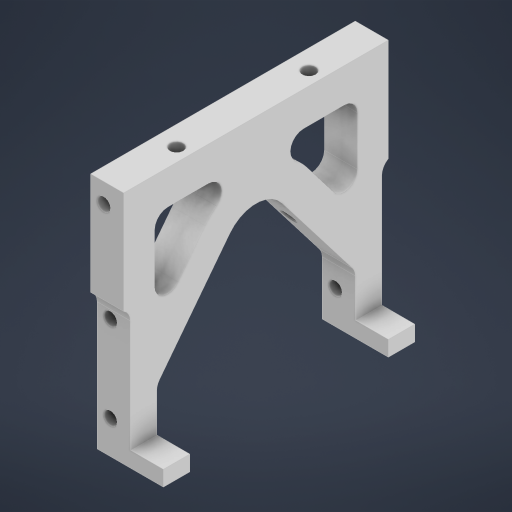
# Autodesk Inventor part: InsidePereborka
Saved by Autodesk Inventor 2024 (Build 280153000, 153)
## iProperties
Created: 2023-01-07
Part Number: InsidePereborka
Material: Типовые
Document SubType Name: Modeling
Designer: KirikDK
Density: 1 g/cm^3
Appearance: По умолчанию
Mass: 27.6494 g
Surface Area: 128.309 cm^2
Volume: 27.6494 cm^3
Author: KirikDK
Autodesk Inventor part; units mm, degrees
ref_plane "YZ Plane" through (0, 0, 0) normal (1, 0, 0) x (0, 1, 0)
ref_plane "XZ Plane" through (0, 0, 0) normal (0, 1, 0) x (-1, 0, 0)
ref_plane "XY Plane" through (0, 0, 0) normal (0, 0, 1) x (1, 0, 0)
sketch "Эскиз1" plane through (0, 0, 0) normal (1, 0, 0) x (0, 1, 0)
  line L0 (49.3333, 18.3333) -> (-26.6667, 18.3333)
  line L1 (-26.6667, 18.3333) -> (-26.6667, -61.6667)
  line L2 (-26.6667, -61.6667) -> (49.3333, -61.6667)
  line L3 (49.3333, -61.6667) -> (49.3333, 18.3333)
  line L4 (17.3333, 18.3333) -> (17.3333, 16.3333)
  line L5 (17.3333, 16.3333) -> (-24.6667, 16.3333)
  line L6 (-24.6667, 16.3333) -> (-24.6667, -21.6667)
  line L7 (-24.6667, -21.6667) -> (-26.6667, -21.6667)
  line L8 (17.3333, -61.6667) -> (17.3333, -59.6667)
  line L9 (17.3333, -59.6667) -> (-24.6667, -59.6667)
  line L10 (-24.6667, -59.6667) -> (-24.6667, -21.6667)
  line L11 (-24.6667, -21.6667) -> (-26.6667, -21.6667)
  line L12 (-24.6667, 8.3333) -> (-7, 8.3333)
  line L13 (-7, 8.3333) -> (-7, -51.6667)
  line L14 (-7, -51.6667) -> (-24.6667, -51.6667)
  line L15 (-24.6667, -51.6667) -> (-24.6667, 8.3333)
  line L16 (-7, 8.3333) -> (32, -21.6667)
  line L17 (32, -21.6667) -> (-7, -51.6667)
  point P0 (0, 0)
  point P1 (-24.6667, -51.6667)
  dimension "d0" = 80
  dimension "d1" = 2
  dimension "d2" = 2
  dimension "d3" = 2
  dimension "d4" = 2
  dimension "d5" = 44
  dimension "d6" = 44
  dimension "d7" = 40
  dimension "d8" = 40
  dimension "d9" = 76
  dimension "d10" = 10
  dimension "d11" = 10
  constraints: 36 end point, 8 perpendicular, 4 parallel, 3 point on line, 2 horizontal, 2 midpoint, 2 vertical
  measures "d0" distance of L2.end L0.start
  measures "d1" distance between parallel lines of L0 L5
  measures "d2" distance between parallel lines of L1 L6
  measures "d3" distance between parallel lines of L1 L10
  measures "d4" distance between parallel lines of L2 L9
  measures "d5" distance between parallel lines of L1 L8
  measures "d6" distance between parallel lines of L1 L4
  measures "d7" distance between parallel lines of L0 L7
  measures "d8" distance between parallel lines of L11 L2
  measures "d9" distance between parallel lines of L1 L3
  measures "d10" distance between parallel lines of L0 L12
  measures "d11" distance between parallel lines of L2 L14
extrude "Выдавливание1" add sketch "Эскиз1" along normal blind 10 contours L3 L2 L8 L9 L10 L14 L17 L16 L12 L6 L5 L4 L0
fillet "Сопряжение1" radius 10 1 edges at (5, 32, -21.6667)
fillet "Сопряжение3" radius 4 4 edges at (5, 17.3333, -59.6667) (5, 17.3333, 16.3333) (5, -7, -51.6667) (5, -7, 8.3333)
sketch "Эскиз2" plane through (10, 49.3333, -61.6667) normal (0, 0, -1) x (-1, 0, 0)
  circle A0 centre (6, -7) radius 2
  circle A1 centre (6, -38) radius 2
  circle A2 centre (6, -64) radius 2
  point P0 (10, -49.3333)
  constraints: 3 centre point
sketch "Эскиз3" plane through (0, 49.3333, 18.3333) normal (0, 1, 0) x (1, 0, 0)
  circle A0 centre (6, 60) radius 2
  circle A1 centre (6, 20) radius 2
  point P0 (0, 18.3333)
  constraints: 2 centre point
extrude "Выдавливание2" cut sketch "Эскиз2" against normal blind 100
extrude "Выдавливание3" cut sketch "Эскиз3" against normal blind 20
sketch "Эскиз4" plane through (10, 0, 0) normal (1, 0, 0) x (0, 0, -1)
  line L0 (59.6667, -24.6667) -> (59.6667, 13.8692) projected
  arc A0 (61.6667, 17.3333) -> (59.6667, 13.8692) centre (63.6667, 13.8692) ccw projected
  line L1 (61.6667, 17.3333) -> (61.6667, 49.3333) projected
  line L2 (61.6667, 49.3333) -> (-18.3333, 49.3333) projected
  line L3 (-18.3333, 49.3333) -> (-18.3333, 17.3333) projected
  arc A1 (-16.3333, 13.8692) -> (-18.3333, 17.3333) centre (-20.3333, 13.8692) ccw projected
  line L4 (-16.3333, 13.8692) -> (-16.3333, -24.6667) projected
  line L5 (-16.3333, -24.6667) -> (-8.3333, -24.6667) projected
  line L6 (-8.3333, -24.6667) -> (-8.3333, -8.3605) projected
  arc A2 (-7.5038, -5.9216) -> (-8.3333, -8.3605) centre (-4.3333, -8.3605) ccw projected
  line L7 (-7.5038, -5.9216) -> (13.7404, 21.6959) projected
  arc A3 (29.5929, 21.6959) -> (13.7404, 21.6959) centre (21.6667, 15.5988) ccw projected
  line L8 (29.5929, 21.6959) -> (50.8372, -5.9216) projected
  arc A4 (51.6667, -8.3605) -> (50.8372, -5.9216) centre (47.6667, -8.3605) ccw projected
  line L9 (51.6667, -8.3605) -> (51.6667, -24.6667) projected
  line L10 (51.6667, -24.6667) -> (59.6667, -24.6667) projected
  line L11 (-9, 7.4411) -> (-9, 40)
  line L12 (-9, 40) -> (52.3333, 40)
  line L13 (52.3333, 40) -> (52.3333, 7.4411)
  line L14 (52.3333, 7.4411) -> (36.9907, 27.3865)
  arc A5 (36.9907, 27.3865) -> (6.3426, 27.3865) centre (21.6667, 15.5988) ccw
  line L15 (6.3426, 27.3865) -> (-9, 7.4411)
  point P0 (0, 0)
  constraints: 10 end point, 2 point on circle, 1 centre point, 5 other
extrude "Выдавливание4" cut sketch "Эскиз4" against normal blind 22 contours L11 L12 L13 L14 A5 L15
sketch "Эскиз5" plane through (10, 0, 0) normal (1, 0, 0) x (0, 0, -1)
  line L0 (11.6667, 43) -> (31.6667, 43)
  line L1 (31.6667, 43) -> (31.6667, 31)
  line L2 (31.6667, 31) -> (11.6667, 31)
  line L3 (11.6667, 31) -> (11.6667, 43)
  line L4 (61.6667, 17.3333) -> (61.6667, 49.3333) projected
  line L5 (-18.3333, 49.3333) -> (-18.3333, 17.3333) projected
  line L6 (-11, 40) -> (55, 40)
  line L7 (55, 40) -> (55, 38)
  line L8 (55, 38) -> (-11, 38)
  line L9 (-11, 38) -> (-11, 40)
  line L10 (52.3333, 7.4411) -> (44.4016, 17.7523)
  line L11 (52.3333, 7.4411) -> (36.9907, 27.3865) projected
  line L12 (44.4016, 17.7523) -> (41, 14)
  line L13 (41, 14) -> (54.2371, 2)
  line L14 (54.2371, 2) -> (54.6936, 25.6036)
  line L15 (54.6936, 25.6036) -> (52.3333, 23)
  line L16 (52.3333, 13.3333) -> (52.3333, 9.3333) projected
  line L17 (52.3333, 40) -> (52.3333, 7.4411) projected
  line L18 (52.3333, 23) -> (52.3333, 7.4411)
  line L19 (-9, 7.4411) -> (6.3426, 27.3865) projected
  line L20 (1.5689, 21.1808) -> (4, 19)
  line L21 (4, 19) -> (-11, 1.3744)
  line L22 (-11, 1.3744) -> (-11, 26)
  line L23 (-11, 26) -> (-9, 26)
  line L24 (-9, 7.4411) -> (-9, 40) projected
  line L25 (1.5689, 21.1808) -> (-9, 7.4411)
  line L26 (-9, 7.4411) -> (-9, 26)
  point P0 (0, 0)
  point P1 (31.6667, 40)
  point P2 (31.6667, 38)
  point P3 (11.6667, 38)
  point P4 (11.6667, 40)
  dimension "d23" = 30
  dimension "d24" = 30
  constraints: 40 end point, 5 parallel, 5 perpendicular, 3 point on line, 2 horizontal, 1 vertical
  measures "d23" distance between parallel lines of L4 L1
  measures "d24" distance between parallel lines of L5 L3
extrude "Выдавливание5" add sketch "Эскиз5" against normal blind 10
fillet "Сопряжение4" radius 4 8 edges at (5, 38, -52.3333) (5, 38, -11.6667) (5, 32.145, -11.6667) (5, 32.145, -31.6667) (5, 38, -31.6667) (5, 7.4411, -52.3333) (5, 7.4411, 9) (5, 38, 9)
sketch "Эскиз6" plane through (10, 0, 0) normal (1, 0, 0) x (0, 0, -1)
  line L0 (-16.3333, 13.8692) -> (-16.3333, -24.6667) projected
  line L1 (-8.3333, -24.6667) -> (-8.3333, -8.3605) projected
  line L2 (-16.3333, -24.6667) -> (-8.3333, -24.6667)
  line L3 (-8.3333, -24.6667) -> (-8.3333, -20)
  line L4 (-8.3333, -20) -> (-16.3333, -20)
  line L5 (-16.3333, -20) -> (-16.3333, -24.6667)
  line L6 (59.6667, -24.6667) -> (59.6667, 13.8692) projected
  line L7 (51.6667, -8.3605) -> (51.6667, -24.6667) projected
  line L8 (59.6667, -24.6667) -> (51.6667, -24.6667)
  line L9 (51.6667, -24.6667) -> (51.6667, -20)
  line L10 (51.6667, -20) -> (59.6667, -20)
  line L11 (59.6667, -20) -> (59.6667, -24.6667)
  point P0 (0, 0)
  constraints: 16 end point, 4 parallel, 3 point on line, 2 horizontal, 2 perpendicular
extrude "Выдавливание6" add sketch "Эскиз6" along normal blind 10
sketch "Sketch7" plane through (0, 49.3333, 18.3333) normal (0, 1, 0) x (1, 0, 0)
  line L0 (0, 81) -> (10, 81)
  line L1 (10, 81) -> (10, -1)
  line L2 (10, -1) -> (0, -1)
  line L3 (0, -1) -> (0, 81)
  point P0 (0, 18.3333)
  constraints: 8 end point, 2 parallel, 1 horizontal, 1 perpendicular
extrude "Extrusion7" cut sketch "Sketch7" against normal blind 1
